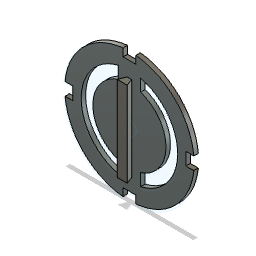
final-lid-threading-space (Autodesk Fusion 360 design; units mm, degrees)
Autodesk Fusion 360 part; units mm, degrees
note: some values were not read from the file. Chosen so that the rebuilt part matches the saved one: which pieces of a blend or face edit are solid. Set by a fixed rule: which sketch regions a step uses.
sketch "Sketch1" plane through (0, 0, 0) normal (0, 0, 1) x (1, 0, 0)
  circle A0 centre (0, 0) radius 28
  dimension "d1" = 56
  constraint coincident A0.centre origin
  measures "d1" diameter of A0
sketch "Sketch2" plane through (0, 0, 0) normal (0, 0, 1) x (1, 0, 0)
sketch "Sketch3" plane through (0, 0, 0) normal (0, 0, 1) x (1, 0, 0)
  circle A0 centre (0, 0) radius 5
  circle A1 centre (0, 17.482745) radius 6
  circle A2 centre (-16.617869, 5.394747) radius 6
  circle A3 centre (-10.266823, -14.146708) radius 6
  circle A4 centre (10.298315, -14.141643) radius 6
  circle A5 centre (16.649932, 5.399061) radius 6
  dimension "d11" = 12
  dimension "d12" = 12
  dimension "d13" = 12
  dimension "d14" = 12
  dimension "d15" = 12
  constraint coincident A0.centre origin
  measures "d11" diameter of A1
  measures "d12" diameter of A2
  measures "d13" diameter of A3
  measures "d14" diameter of A4
  measures "d15" diameter of A5
extrude "Extrude1" add sketch "Sketch3" along normal blind 18 makes body 1 at (16.290857, -14.440718, 12) makes body 2 at (5.992542, 17.18367, 12) makes body 3 at (22.642473, 5.099985, 12) makes body 4 at (-4.274281, -14.445784, 12) makes body 5 at (-10.625328, 5.095671, 12) makes body 6 at (4.993785, -0.249229, 12)
extrude "Extrude2" add sketch "Sketch1" against normal blind 5 bodies 1 2 3 4 5 6
extrude "Extrude3" cut 6 faces at (-0.119858, 15.883355, 18) (-15.887187, 6.660325, 18) (-1.501615, -0.72314, 18) (-13.649983, -15.403045, 18) (12.100253, -13.870045, 18) (17.521533, 6.714854, 18) along direction (0, 0, -1) blind 32 on bodies 1 bodies 1
extrude "Extrude4" cut 1 faces at (-20.263403, -6.403476, 0) along direction (0, 0, -1) blind 2 on bodies 1 bodies 1
extrude "Extrude5" add 1 faces at (-20.263403, -6.403476, -2) along direction (0, 0, 1) blind 1 on bodies 1 bodies 1
extrude "Extrude6" cut 1 faces at (-20.263403, -6.403476, -1) along direction (0, 0, -1) blind 0.5 on bodies 1 bodies 1
extrude "Extrude7" cut 1 faces at (-20.263403, -6.403476, -1.5) along direction (0, 0, -1) blind 1 on bodies 1 bodies 1
extrude "Extrude8" cut 1 faces at (-20.263403, -6.403476, -2.5) along direction (0, 0, -1) blind 0.5 on bodies 1 bodies 1
sketch "Sketch4" plane through (0, 0, 0) normal (0, 0, 1) x (1, 0, 0)
  circle A0 centre (75.004509, -0.00652) radius 28
  circle A1 centre (75.004509, -0.00652) radius 5
  line L0 (75.004509, -0.00652) -> (103, -0.00652) construction
  line L1 (75.004509, 7.928105) -> (71.001656, 22.993491)
  line L2 (71.001656, 22.993491) -> (79.004454, 22.993491)
  line L3 (79.004454, 22.993491) -> (75.004509, 7.928105)
  line L4 (68.132923, -3.973832) -> (53.002764, -7.794084)
  line L5 (68.132923, -3.973832) -> (57.4732, -15.370601)
  line L6 (53.002764, -7.794084) -> (57.4732, -15.370601)
  line L7 (81.876096, -3.973832) -> (92.79521, -15.122329)
  line L8 (81.876096, -3.973832) -> (96.990535, -7.855813)
  line L9 (96.990535, -7.855813) -> (92.79521, -15.122329)
  dimension "d32" = 56
  dimension "d33" = 10
  dimension "d38" = 15.605
  dimension "d39" = 15.605
  dimension "d40" = 15.605
  dimension "d41" = 15.605
  constraint concentric A0 A1
  constraint horizontal L0
  measures "d32" diameter of A0
  measures "d33" diameter of A1
extrude "Extrude9" add sketch "Sketch4" along normal blind 2 separate body makes body 7
sketch "Sketch5" plane through (0, 0, 0) normal (0, 0, 1) x (1, 0, 0)
  circle A0 centre (-75, 0) radius 28
  circle A1 centre (-75, 0) radius 3
  circle A2 centre (-75, 0) radius 28
  line L0 (-75, 0) -> (-75, 28)
  line L1 (-75, 0) -> (-46.346903, 0) construction
  line L2 (-75, 0) -> (-82.246933, 27.045923)
  line L3 (-75, 0) -> (-47, 0) construction
  line L4 (-75, 0) -> (-67.753067, 27.045923)
  line L5 (-75, 0) -> (-47, 0) construction
  line L6 (-75, 0) -> (-102.045923, 7.246933)
  line L7 (-75, 0) -> (-47, 0) construction
  line L8 (-75, 0) -> (-47.954077, 7.246933)
  line L9 (-75, 0) -> (-47, 0) construction
  line L10 (-47.954077, 7.246933) -> (-102.045923, -7.246933)
  line L11 (-102.045923, 7.246933) -> (-47.954077, -7.246933)
  line L12 (-67.753067, 27.045923) -> (-82.246933, -27.045923)
  line L13 (-82.246933, 27.045923) -> (-67.753067, -27.045923)
  circle A3 centre (-75, 0) radius 17.043974
  circle A4 centre (-75, 0) radius 23
  line L14 (-50.18569, -14.326549) -> (-99.26887, 13.965025)
  line L15 (-99.248711, -14) -> (-50.73113, 13.965025)
  line L16 (-75, 0) -> (-94.79899, -19.79899)
  line L17 (-75, 0) -> (-47, 0) construction
  line L18 (-75, 0) -> (-55.20101, -19.79899)
  line L19 (-75, 0) -> (-47, 0) construction
  dimension "d44" = 56
  dimension "d45" = 6
  dimension "d47" = 28
  dimension "d48" = 28.653097
  dimension "d50" = 105
  dimension "d51" = 28
  dimension "d52" = 75
  dimension "d53" = 28
  dimension "d54" = 165
  dimension "d55" = 28
  dimension "d56" = 15
  dimension "d57" = 28
  dimension "d58" = 135
  dimension "d59" = 28
  dimension "d60" = 45
  dimension "d61" = 28
  constraint concentric A0 A1
  constraint concentric A0 A2
  constraint coincident A0.centre A1.centre
  constraint coincident A0 L0.end
  constraint vertical L0
  constraint horizontal L1
  constraint horizontal L3
  constraint horizontal L5
  constraint horizontal L7
  constraint horizontal L9
  constraint parallel L8 L10
  constraint parallel L6 L11
  constraint perpendicular L11 L12
  constraint parallel L2 L13
  constraint concentric A2 A3
  constraint horizontal L17
  constraint horizontal L19
  measures "d44" diameter of A0
  measures "d45" diameter of A1
  measures "d50" angle of L2 L3
  measures "d52" angle of L4 L5
  measures "d54" angle of L6 L7
  measures "d56" angle of L8 L9
  measures "d58" angle of L16 L17
  measures "d60" angle of L18 L19
extrude "Extrude10" add sketch "Sketch5" along normal blind 2 separate body contours A0 A2 L8 L10 L11 A4 | A0 A2 L8 L10 A4 L15 | A0 A2 L11 A4 L14 | A0 A2 L4 L12 A4 L15 | A0 A2 A4 L14 L18 | L11 A3 A4 L14 | A0 A2 L0 L4 L12 A4 | A1 L8 L10 L11 A3 | A1 L8 L10 A3 L15 | A0 A2 L13 A4 L18 | A3 A4 L14 L18 | A1 L11 A3 L14 | A0 A2 L0 L2 L13 A4 | L0 L4 L12 A3 A4 | A1 L4 L12 A3 L15 | A0 A2 L12 L13 A4 | A1 A3 L14 L18 | A0 A2 L2 L13 A4 L14 | L0 L2 L13 A3 A4 | A1 L0 L4 L12 A3 | A0 A2 L12 A4 L16 | A1 L13 A3 L18 | A0 A2 L6 L11 A4 L14 | A1 L0 L2 L13 A3 | A0 A2 A4 L15 L16 | A1 L12 L13 A3 | A0 A2 L6 L10 L11 A4 | A1 L2 L13 A3 L14 | A0 A2 L10 A4 L15 | A3 A4 L15 L16 | A1 L12 A3 L16 | A1 L6 L11 A3 L14 | A1 L6 L10 L11 A3 | A1 L10 A3 L15 | L10 A3 A4 L15 | A1 A3 L15 L16 picked at (-48.731357, -1.481648) picked at (-51.80207, 12.414029) picked at (-51.510363, -11.852216) picked at (-53.410337, 14.986946) picked at (-52.632957, -13.854762) picked at (-56.26491, -9.478078) picked at (-71.897636, 26.126849) picked at (-62.951324, -2.715806) picked at (-64.052626, 5.719309) picked at (-58.051392, -20.08667) picked at (-57.162699, -11.075699) picked at (-64.028373, -5.672044) picked at (-76.481648, 26.268643) picked at (-73.836646, 20.963865) picked at (-64.764526, 6.88652) picked at (-70.36541, -25.86987) picked at (-64.565431, -6.608497) picked at (-96.58967, 14.986937) picked at (-79.786017, 20.443362) picked at (-72.369365, 12.067558) picked at (-91.948608, -20.08667) picked at (-66.915364, -9.317954) picked at (-98.197937, 12.414017) picked at (-76.568867, 12.250913) picked at (-97.36725, -13.854421) picked at (-75.741562, -12.314045) picked at (-100.86987, -4.63459) picked at (-85.235539, 6.886427) picked at (-98.489798, -11.851903) picked at (-92.837488, -11.075391) picked at (-80.397495, -11.09291) picked at (-85.947432, 5.719204) picked at (-87.086384, -2.470816) picked at (-85.971749, -5.671808) picked at (-93.735235, -9.477795) picked at (-85.434723, -6.608247) makes body 8
sketch "Sketch8" plane through (0, 0, 0) normal (0, 0, 1) x (1, 0, 0)
  circle A0 centre (-165, 0) radius 28
  line L0 (-189.512038, 2.74198) -> (-196.487957, 2.74198)
  line L1 (-196.487957, 2.74198) -> (-196.487957, -2.764168)
  line L2 (-196.487957, -2.764168) -> (-189.512038, -2.764168)
  line L3 (-189.512038, -2.764168) -> (-189.512038, 2.74198)
  line L4 (-189.512038, 2.74198) -> (-196.487957, -2.764168) construction
  line L5 (-196.487957, 2.74198) -> (-189.512038, -2.764168) construction
  line L6 (-140.547399, 2.726991) -> (-133.452644, 2.726991)
  line L7 (-133.452644, 2.726991) -> (-133.452644, -2.796303)
  line L8 (-133.452644, -2.796303) -> (-140.547399, -2.796303)
  line L9 (-140.547399, -2.796303) -> (-140.547399, 2.726991)
  line L10 (-140.547399, 2.726991) -> (-133.452644, -2.796303) construction
  line L11 (-133.452644, 2.726991) -> (-140.547399, -2.796303) construction
  line L12 (-167.752196, 31.487615) -> (-162.247804, 31.487615)
  line L13 (-162.247804, 31.487615) -> (-162.247804, 24.512385)
  line L14 (-162.247804, 24.512385) -> (-167.752196, 24.512385)
  line L15 (-167.752196, 24.512385) -> (-167.752196, 31.487615)
  line L16 (-167.752196, 31.487615) -> (-162.247804, 24.512385) construction
  line L17 (-162.247804, 31.487615) -> (-167.752196, 24.512385) construction
  line L18 (-167.749074, -24.505866) -> (-162.250926, -24.505866)
  line L19 (-162.250926, -24.505866) -> (-162.250926, -31.494134)
  line L20 (-162.250926, -31.494134) -> (-167.749074, -31.494134)
  line L21 (-167.749074, -31.494134) -> (-167.749074, -24.505866)
  line L22 (-167.749074, -24.505866) -> (-162.250926, -31.494134) construction
  line L23 (-162.250926, -24.505866) -> (-167.749074, -31.494134) construction
  point P0 (-192.999998, -0.011094)
  point P1 (-137.000021, -0.034656)
  point P2 (-165, 28)
  point P3 (-165, -28)
  dimension "d71" = 56
  constraint horizontal L0
  constraint perpendicular L0 L1
  constraint parallel L0 L2
  constraint parallel L1 L3
  constraint horizontal L6
  constraint perpendicular L6 L7
  constraint parallel L6 L8
  constraint parallel L7 L9
  constraint horizontal L12
  constraint perpendicular L12 L13
  constraint parallel L12 L14
  constraint parallel L13 L15
  constraint coincident L16 P2
  constraint coincident L17 P2
  constraint coincident A0 P2
  constraint horizontal L18
  constraint perpendicular L18 L19
  constraint parallel L18 L20
  constraint parallel L19 L21
  constraint coincident L22 P3
  constraint coincident L23 P3
  constraint coincident A0 P3
  measures "d71" diameter of A0
sketch "Sketch9" plane through (0, 0, 0) normal (0, 0, 1) x (1, 0, 0)
  circle A0 centre (-165.000002, 0) radius 20.880613
  circle A1 centre (-165.000002, 0) radius 15.811389
  line L0 (-169.838066, 20.312389) -> (-169.838066, 15.053011)
  line L1 (-160.161939, 20.312389) -> (-160.161939, 15.053011)
  line L2 (-169.84149, -15.051911) -> (-169.84149, -20.311573)
  line L3 (-169.84149, -20.311573) -> (-169.84149, -15.051911)
  line L4 (-160.158515, -15.051911) -> (-160.158515, -20.311573)
  constraint concentric A0 A1
  constraint vertical L0
  constraint parallel L0 L1
  constraint parallel L1 L2
  constraint parallel L3 L4
extrude "Extrude11" add sketch "Sketch8" along normal blind 2 separate body contours A0 L0 L2 L3 L6 L8 L9 L13 L14 L15 L18 L19 L21 picked at (-165.93617, -8.181014) makes body 9
extrude "Extrude12" cut sketch "Sketch9" along normal blind 5 contours A0 A1 L1 L4 | A0 A1 L0 L2 L3 picked at (-159.177578, 18.246004) picked at (-184.099632, 1.422042) bodies 9
sketch "Sketch10" plane through (0, 0, 2) normal (0, 0, 1) x (1, 0, 0)
  arc A0 (-160.158515, -15.051911) -> (-160.161939, 15.053011) centre (-165.000002, 0) ccw
  line L0 (-160.161939, 15.053011) -> (-160.161939, 20.312389)
  arc A1 (-160.158515, -20.311573) -> (-160.161939, 20.312389) centre (-165.000002, 0) ccw
  line L1 (-160.158515, -20.311573) -> (-160.158515, -15.051911)
  line L2 (-169.838066, 20.312389) -> (-169.838066, 15.053011)
  arc A2 (-169.838066, 15.053011) -> (-169.84149, -15.051911) centre (-165.000002, 0) ccw
  line L3 (-169.84149, -15.051911) -> (-169.84149, -20.311573)
  arc A3 (-169.838066, 20.312389) -> (-169.84149, -20.311573) centre (-165.000002, 0) ccw
  line L4 (-189.512038, -2.764168) -> (-192.863226, -2.764168)
  arc A4 (-192.863226, -2.764168) -> (-167.749074, -27.864719) centre (-165, 0) ccw
  line L5 (-167.749074, -27.864719) -> (-167.749074, -24.505866)
  line L6 (-167.749074, -24.505866) -> (-162.250926, -24.505866)
  line L7 (-162.250926, -24.505866) -> (-162.250926, -27.864719)
  arc A5 (-162.250926, -27.864719) -> (-137.13998, -2.796303) centre (-165, 0) ccw
  line L8 (-137.13998, -2.796303) -> (-140.547399, -2.796303)
  line L9 (-140.547399, -2.796303) -> (-140.547399, 2.726991)
  line L10 (-140.547399, 2.726991) -> (-137.133111, 2.726991)
  arc A6 (-137.133111, 2.726991) -> (-162.247804, 27.864411) centre (-165, 0) ccw
  line L11 (-162.247804, 27.864411) -> (-162.247804, 24.512385)
  line L12 (-162.247804, 24.512385) -> (-167.752196, 24.512385)
  line L13 (-167.752196, 24.512385) -> (-167.752196, 27.864411)
  arc A7 (-167.752196, 27.864411) -> (-192.865418, 2.74198) centre (-165, 0) ccw
  line L14 (-192.865418, 2.74198) -> (-189.512038, 2.74198)
  line L15 (-189.512038, 2.74198) -> (-189.512038, -2.764168)
  circle A8 centre (-165.000002, 0) radius 3
  dimension "d76" = 6
  constraint concentric A0 A8
  measures "d76" diameter of A8
extrude "Extrude13" cut sketch "Sketch10" against normal blind 4 contours A8 picked at (-163.931471, 0.781831) bodies 9
scale "Scale1" factors (1, 1, 1) about (-160.161939, 20.312389, 2) bodies 9
sketch "Sketch11" plane through (0, 0, 2) normal (0, 0, 1) x (1, 0, 0)
  circle A0 centre (-165.000002, 0) radius 3
  arc A1 (-160.158515, -15.051911) -> (-160.161939, 15.053011) centre (-165.000002, 0) ccw
  line L0 (-160.161939, 15.053011) -> (-160.161939, 20.312389)
  arc A2 (-160.158515, -20.311573) -> (-160.161939, 20.312389) centre (-165.000002, 0) ccw
  line L1 (-160.158515, -20.311573) -> (-160.158515, -15.051911)
  line L2 (-169.838066, 20.312389) -> (-169.838066, 15.053011)
  arc A3 (-169.838066, 15.053011) -> (-169.84149, -15.051911) centre (-165.000002, 0) ccw
  line L3 (-169.84149, -15.051911) -> (-169.84149, -20.311573)
  arc A4 (-169.838066, 20.312389) -> (-169.84149, -20.311573) centre (-165.000002, 0) ccw
  line L4 (-189.512038, -2.764168) -> (-192.863226, -2.764168)
  arc A5 (-192.863226, -2.764168) -> (-167.749074, -27.864719) centre (-165, 0) ccw
  line L5 (-167.749074, -27.864719) -> (-167.749074, -24.505866)
  line L6 (-167.749074, -24.505866) -> (-162.250926, -24.505866)
  line L7 (-162.250926, -24.505866) -> (-162.250926, -27.864719)
  arc A6 (-162.250926, -27.864719) -> (-137.13998, -2.796303) centre (-165, 0) ccw
  line L8 (-137.13998, -2.796303) -> (-140.547399, -2.796303)
  line L9 (-140.547399, -2.796303) -> (-140.547399, 2.726991)
  line L10 (-140.547399, 2.726991) -> (-137.133111, 2.726991)
  arc A7 (-137.133111, 2.726991) -> (-162.247804, 27.864411) centre (-165, 0) ccw
  line L11 (-162.247804, 27.864411) -> (-162.247804, 24.512385)
  line L12 (-162.247804, 24.512385) -> (-167.752196, 24.512385)
  line L13 (-167.752196, 24.512385) -> (-167.752196, 27.864411)
  arc A8 (-167.752196, 27.864411) -> (-192.865418, 2.74198) centre (-165, 0) ccw
  line L14 (-192.865418, 2.74198) -> (-189.512038, 2.74198)
  line L15 (-189.512038, 2.74198) -> (-189.512038, -2.764168)
scale "Scale3" factors (0.98, 0.98, 0.95) about (-162.247804, 24.512385, 2) bodies 9
sketch "Sketch12" plane through (0, 0, 2) normal (0, 0, 1) x (1, 0, 0)
  line L0 (-167.000002, 19) -> (-162.585447, 19)
  line L1 (-162.585447, 19) -> (-162.585447, 17.057661)
  line L2 (-162.585447, 17.057661) -> (-167.000002, 17.057661)
  line L3 (-167.000002, 17.057661) -> (-167.000002, 19)
  line L4 (-167.000002, -16) -> (-162.585447, -16)
  line L5 (-162.585447, -16) -> (-162.585447, -17.887993)
  line L6 (-162.585447, -17.887993) -> (-167.000002, -17.887993)
  line L7 (-167.000002, -17.887993) -> (-167.000002, -16)
  constraint horizontal L0
  constraint vertical L1
  constraint horizontal L2
  constraint vertical L3
  constraint horizontal L4
  constraint vertical L5
  constraint horizontal L6
  constraint vertical L7
extrude "Extrude14" add sketch "Sketch12" along normal blind 4 bodies 9
sketch "Sketch13" plane through (0, 0, 6) normal (0, 0, 1) x (1, 0, 0)
  line L0 (-167.000002, 17.057661) -> (-162.585447, 17.057661)
  line L1 (-162.585447, 17.057661) -> (-162.585447, 19)
  line L2 (-162.585447, 19) -> (-167.000002, 19)
  line L3 (-167.000002, 19) -> (-167.000002, 17.057661)
  line L4 (-167.000002, 19) -> (-162.585447, 19)
  line L5 (-162.585447, 19) -> (-162.585447, -17.933136)
  line L6 (-162.585447, -17.933136) -> (-167.000002, -17.933136)
  line L7 (-167.000002, -17.933136) -> (-167.000002, 19)
  constraint horizontal L4
  constraint vertical L5
  constraint horizontal L6
  constraint vertical L7
extrude "Extrude15" add sketch "Sketch13" along normal blind 1 bodies 9
fillet "Fillet1" radius 1.5 1 edges at (-164.792725, 19, 7) on bodies 9
fillet "Fillet2" radius 1.5 1 edges at (-164.792725, -17.933136, 7) on bodies 9
delete_face "DeleteFace1" 1 faces at (-165.528484, 6.160359, 7) on bodies 9
delete_face "DeleteFace2" 1 faces at (-162.585447, 17.705107, 4.5) on bodies 9
delete_face "DeleteFace3" 1 faces at (-162.585447, -17.258662, 4.666667) on bodies 9
sketch "Sketch14" plane through (0, 0, 0.1) normal (0, 0, -1) x (-1, 0, 0)
  circle A0 centre (164.944958, 0.490248) radius 2.94
  arc A1 (160.203656, 15.242199) -> (160.200301, -14.260625) centre (164.944958, 0.490248) ccw
  line L0 (160.200301, -14.260625) -> (160.200301, -19.415094)
  arc A2 (160.203656, 20.396389) -> (160.200301, -19.415094) centre (164.944958, 0.490248) ccw
  line L1 (160.203656, 20.396389) -> (160.203656, 15.242199)
  line L2 (169.686261, 15.242199) -> (169.686261, 20.396389)
  arc A3 (169.689616, -19.415094) -> (169.686261, 20.396389) centre (164.944958, 0.490248) ccw
  line L3 (169.689616, -19.415094) -> (169.689616, -14.260625)
  arc A4 (169.689616, -14.260625) -> (169.686261, 15.242199) centre (164.944958, 0.490248) ccw
  line L4 (192.250918, -2.218637) -> (188.966754, -2.218637)
  line L5 (188.966754, -2.218637) -> (188.966754, 3.177388)
  line L6 (188.966754, 3.177388) -> (192.253066, 3.177388)
  arc A5 (192.253066, 3.177388) -> (167.642108, 27.797371) centre (164.944956, 0.490248) ccw
  line L7 (167.642108, 27.797371) -> (167.642108, 24.512385)
  line L8 (167.642108, 24.512385) -> (162.247804, 24.512385)
  line L9 (162.247804, 24.512385) -> (162.247804, 27.797371)
  arc A6 (162.247804, 27.797371) -> (137.635405, 3.162699) centre (164.944956, 0.490248) ccw
  line L10 (137.635405, 3.162699) -> (140.981407, 3.162699)
  line L11 (140.981407, 3.162699) -> (140.981407, -2.250129)
  line L12 (140.981407, -2.250129) -> (137.642137, -2.250129)
  arc A7 (137.642137, -2.250129) -> (162.250864, -26.817177) centre (164.944956, 0.490248) ccw
  line L13 (162.250864, -26.817177) -> (162.250864, -23.525501)
  line L14 (162.250864, -23.525501) -> (167.639049, -23.525501)
  line L15 (167.639049, -23.525501) -> (167.639049, -26.817177)
  arc A8 (167.639049, -26.817177) -> (192.250918, -2.218637) centre (164.944956, 0.490248) ccw
  circle A9 centre (164.944958, 0.490248) radius 3.609399
  constraint concentric A0 A9
extrude "Extrude16" add sketch "Sketch14" against normal blind 1.9 contours A0 | A9 picked at (167.136053, 0.636309) picked at (165.870305, 3.73861) bodies 9
sketch "Sketch15" plane through (0, 0, 2) normal (0, 0, 1) x (1, 0, 0)
  line L0 (-166.000002, 18) -> (-164.000002, 18)
  line L1 (-164.000002, 18) -> (-164.000002, -18)
  line L2 (-164.000002, -18) -> (-166.000002, -18)
  line L3 (-166.000002, -18) -> (-166.000002, 18)
  line L4 (-166.000002, 18) -> (-164.000002, -18) construction
  line L5 (-164.000002, 18) -> (-166.000002, -18) construction
  point P0 (-165.000002, 0)
  constraint horizontal L0
  constraint perpendicular L0 L1
  constraint parallel L0 L2
  constraint parallel L1 L3
extrude "Extrude17" add sketch "Sketch15" along normal blind 3 bodies 9
sketch "Sketch16" plane through (0, 18, 0) normal (0, 1, 0) x (-1, 0, 0)
  line L0 (164.000002, 2) -> (166.000002, 2)
  line L1 (166.000002, 2) -> (166.000002, 5)
  line L2 (166.000002, 5) -> (164.000002, 5)
  line L3 (164.000002, 5) -> (164.000002, 2)
  line L4 (166.000002, 2) -> (167.100002, 5)
  line L5 (167.100002, 5) -> (166.000002, 5)
  line L6 (164.000002, 5) -> (162.899996, 5)
  line L7 (162.899996, 5) -> (164.000002, 2)
  dimension "d98" = 1.1
  dimension "d99" = 1.100006
  constraint perpendicular L1 L5
  constraint perpendicular L3 L6
extrude "Extrude18" add sketch "Sketch16" against normal blind 36 bodies 9
hidden bodies 1 7 8
